inside encoder (Autodesk Fusion 360 design; units mm, degrees)
Autodesk Fusion 360 part; units mm, degrees
note: some values were not read from the file. Set by a fixed rule: which sketch regions a step uses.
(part 1 of 2)
sketch "Sketch1" plane through (0, -20.5, -1.25) normal (0, 0, -1) x (1, 0, 0)
  circle A0 centre (0, -20.5) radius 3
  spline S0 degree 5 poles (-12.6425, -33.7593) (-12.6317, -33.756) (-12.6102, -33.7493) (-12.5779, -33.7393) (-12.535, -33.7257) (-12.4816, -33.7085) (-12.4284, -33.6909) (-12.3754, -33.673) (-12.3227, -33.6548) (-12.2702, -33.6363) (-12.2179, -33.6175) (-12.1659, -33.5983) (-12.114, -33.5788) (-12.0625, -33.5591) (-12.0112, -33.5389) (-11.9601, -33.5185) (-11.9093, -33.4978) (-11.8587, -33.4767) (-11.8084, -33.4553) (-11.7584, -33.4335) (-11.7086, -33.4114) (-11.6591, -33.389) (-11.6099, -33.3662) (-11.561, -33.3431) (-11.5124, -33.3196) (-11.4641, -33.2958) (-11.4161, -33.2716) (-11.3684, -33.2471) (-11.321, -33.2222) (-11.274, -33.1969) (-11.2273, -33.1713) (-11.1809, -33.1453) (-11.1349, -33.1188) (-11.0893, -33.092) (-11.0441, -33.0647) (-10.9992, -33.0371) (-10.9547, -33.009) (-10.9107, -32.9805) (-10.867, -32.9516) (-10.8239, -32.9222) (-10.7812, -32.8923) (-10.739, -32.8619) (-10.6974, -32.8309) (-10.6565, -32.7993) (-10.6161, -32.7671) (-10.5765, -32.7343) (-10.5452, -32.7076) (-10.5221, -32.6872) (-10.5068, -32.6735) (-10.4992, -32.6667) knots -1 -1 -1 -1 -1 -1 -0.977778 -0.955556 -0.933333 -0.911111 -0.888889 -0.866667 -0.844444 -0.822222 -0.8 -0.777778 -0.755556 -0.733333 -0.711111 -0.688889 -0.666667 -0.644444 -0.622222 -0.6 -0.577778 -0.555556 -0.533333 -0.511111 -0.488889 -0.466667 -0.444444 -0.422222 -0.4 -0.377778 -0.355556 -0.333333 -0.311111 -0.288889 -0.266667 -0.244444 -0.222222 -0.2 -0.177778 -0.155556 -0.133333 -0.111111 -0.088889 -0.066667 -0.044444 -0.022222 0 0 0 0 0 0
  arc A1 (-10.4992, -32.6667) -> (-9.4419, -33.5043) centre (0, -20.5) ccw
  spline S1 degree 5 poles (-9.4419, -33.5043) (-9.4469, -33.5133) (-9.4567, -33.5313) (-9.4712, -33.5584) (-9.4901, -33.5949) (-9.513, -33.6411) (-9.5351, -33.6877) (-9.5565, -33.7348) (-9.5772, -33.7824) (-9.5971, -33.8304) (-9.6165, -33.8788) (-9.6352, -33.9275) (-9.6534, -33.9766) (-9.671, -34.026) (-9.6882, -34.0757) (-9.7048, -34.1257) (-9.721, -34.176) (-9.7367, -34.2266) (-9.7519, -34.2774) (-9.7666, -34.3285) (-9.7809, -34.3798) (-9.7947, -34.4314) (-9.8081, -34.4832) (-9.8211, -34.5352) (-9.8337, -34.5875) (-9.8458, -34.64) (-9.8575, -34.6927) (-9.8688, -34.7456) (-9.8797, -34.7987) (-9.8903, -34.852) (-9.9004, -34.9055) (-9.9101, -34.9591) (-9.9194, -35.013) (-9.9284, -35.0671) (-9.937, -35.1213) (-9.9452, -35.1757) (-9.953, -35.2302) (-9.9605, -35.285) (-9.9676, -35.3398) (-9.9743, -35.3949) (-9.9807, -35.4501) (-9.9867, -35.5055) (-9.9923, -35.561) (-9.9976, -35.6166) (-10.0026, -35.6724) (-10.0072, -35.7283) (-10.0106, -35.7732) (-10.0129, -35.8069) (-10.0145, -35.8294) (-10.0152, -35.8407) knots 0 0 0 0 0 0 0.022222 0.044444 0.066667 0.088889 0.111111 0.133333 0.155556 0.177778 0.2 0.222222 0.244444 0.266667 0.288889 0.311111 0.333333 0.355556 0.377778 0.4 0.422222 0.444444 0.466667 0.488889 0.511111 0.533333 0.555556 0.577778 0.6 0.622222 0.644444 0.666667 0.688889 0.711111 0.733333 0.755556 0.777778 0.8 0.822222 0.844444 0.866667 0.888889 0.911111 0.933333 0.955556 0.977778 1 1 1 1 1 1
  arc A2 (-10.0152, -35.8407) -> (-9.6095, -36.098) centre (0, -20.5) ccw
  spline S2 degree 5 poles (-9.6095, -36.098) (-9.5996, -36.0926) (-9.5799, -36.0816) (-9.5504, -36.0651) (-9.5113, -36.0429) (-9.4627, -36.0149) (-9.4143, -35.9866) (-9.3662, -35.9581) (-9.3184, -35.9294) (-9.2709, -35.9003) (-9.2236, -35.8711) (-9.1767, -35.8415) (-9.1301, -35.8117) (-9.0838, -35.7816) (-9.0377, -35.7513) (-8.992, -35.7207) (-8.9466, -35.6898) (-8.9016, -35.6587) (-8.8568, -35.6273) (-8.8124, -35.5956) (-8.7683, -35.5636) (-8.7246, -35.5314) (-8.6812, -35.4989) (-8.6382, -35.4661) (-8.5955, -35.4331) (-8.5532, -35.3997) (-8.5113, -35.3661) (-8.4697, -35.3322) (-8.4286, -35.298) (-8.3878, -35.2635) (-8.3474, -35.2287) (-8.3075, -35.1936) (-8.268, -35.1581) (-8.229, -35.1224) (-8.1904, -35.0864) (-8.1523, -35.05) (-8.1146, -35.0133) (-8.0774, -34.9763) (-8.0407, -34.9389) (-8.0046, -34.9012) (-7.9691, -34.8631) (-7.9341, -34.8245) (-7.8999, -34.7856) (-7.8664, -34.7462) (-7.8337, -34.7063) (-7.8017, -34.6659) (-7.7767, -34.6333) (-7.7583, -34.6086) (-7.7462, -34.592) (-7.7402, -34.5837) knots -1 -1 -1 -1 -1 -1 -0.977778 -0.955556 -0.933333 -0.911111 -0.888889 -0.866667 -0.844444 -0.822222 -0.8 -0.777778 -0.755556 -0.733333 -0.711111 -0.688889 -0.666667 -0.644444 -0.622222 -0.6 -0.577778 -0.555556 -0.533333 -0.511111 -0.488889 -0.466667 -0.444444 -0.422222 -0.4 -0.377778 -0.355556 -0.333333 -0.311111 -0.288889 -0.266667 -0.244444 -0.222222 -0.2 -0.177778 -0.155556 -0.133333 -0.111111 -0.088889 -0.066667 -0.044444 -0.022222 0 0 0 0 0 0
  arc A3 (-7.7402, -34.5837) -> (-6.5319, -35.1832) centre (0, -20.5) ccw
  spline S3 degree 5 poles (-6.5319, -35.1832) (-6.5348, -35.193) (-6.5407, -35.2127) (-6.5493, -35.2422) (-6.5602, -35.2819) (-6.5729, -35.3318) (-6.5849, -35.382) (-6.596, -35.4325) (-6.6063, -35.4833) (-6.6159, -35.5344) (-6.6247, -35.5858) (-6.6329, -35.6374) (-6.6405, -35.6892) (-6.6475, -35.7412) (-6.6539, -35.7934) (-6.6598, -35.8457) (-6.6652, -35.8983) (-6.67, -35.951) (-6.6743, -36.0038) (-6.6781, -36.0569) (-6.6814, -36.1101) (-6.6842, -36.1634) (-6.6865, -36.2169) (-6.6884, -36.2705) (-6.6898, -36.3242) (-6.6908, -36.3781) (-6.6913, -36.432) (-6.6914, -36.4861) (-6.691, -36.5403) (-6.6902, -36.5946) (-6.689, -36.6491) (-6.6873, -36.7036) (-6.6853, -36.7582) (-6.6828, -36.813) (-6.6799, -36.8678) (-6.6766, -36.9227) (-6.6729, -36.9777) (-6.6689, -37.0328) (-6.6644, -37.0879) (-6.6595, -37.1432) (-6.6543, -37.1985) (-6.6486, -37.2539) (-6.6426, -37.3094) (-6.6362, -37.3649) (-6.6295, -37.4205) (-6.6223, -37.4762) (-6.6163, -37.5208) (-6.6117, -37.5542) (-6.6085, -37.5766) (-6.6068, -37.5877) knots 0 0 0 0 0 0 0.022222 0.044444 0.066667 0.088889 0.111111 0.133333 0.155556 0.177778 0.2 0.222222 0.244444 0.266667 0.288889 0.311111 0.333333 0.355556 0.377778 0.4 0.422222 0.444444 0.466667 0.488889 0.511111 0.533333 0.555556 0.577778 0.6 0.622222 0.644444 0.666667 0.688889 0.711111 0.733333 0.755556 0.777778 0.8 0.822222 0.844444 0.866667 0.888889 0.911111 0.933333 0.955556 0.977778 1 1 1 1 1 1
  arc A4 (-6.6068, -37.5877) -> (-6.1565, -37.7551) centre (0, -20.5) ccw
  spline S4 degree 5 poles (-6.1565, -37.7551) (-6.148, -37.7477) (-6.131, -37.7329) (-6.1056, -37.7106) (-6.0719, -37.6807) (-6.0301, -37.6432) (-5.9887, -37.6056) (-5.9476, -37.5677) (-5.9068, -37.5296) (-5.8664, -37.4913) (-5.8263, -37.4529) (-5.7865, -37.4142) (-5.7471, -37.3753) (-5.708, -37.3363) (-5.6693, -37.297) (-5.631, -37.2576) (-5.593, -37.218) (-5.5554, -37.1781) (-5.5181, -37.1381) (-5.4813, -37.0979) (-5.4448, -37.0575) (-5.4087, -37.0169) (-5.3731, -36.9761) (-5.3378, -36.9351) (-5.3029, -36.8938) (-5.2685, -36.8524) (-5.2344, -36.8108) (-5.2009, -36.769) (-5.1677, -36.727) (-5.135, -36.6848) (-5.1028, -36.6423) (-5.071, -36.5997) (-5.0397, -36.5568) (-5.009, -36.5138) (-4.9787, -36.4705) (-4.949, -36.427) (-4.9198, -36.3833) (-4.8911, -36.3393) (-4.863, -36.2951) (-4.8355, -36.2507) (-4.8087, -36.206) (-4.7825, -36.1611) (-4.7571, -36.1159) (-4.7326, -36.0704) (-4.7088, -36.0246) (-4.6859, -35.9784) (-4.6683, -35.9413) (-4.6554, -35.9133) (-4.6471, -35.8946) (-4.6429, -35.8852) knots -1 -1 -1 -1 -1 -1 -0.977778 -0.955556 -0.933333 -0.911111 -0.888889 -0.866667 -0.844444 -0.822222 -0.8 -0.777778 -0.755556 -0.733333 -0.711111 -0.688889 -0.666667 -0.644444 -0.622222 -0.6 -0.577778 -0.555556 -0.533333 -0.511111 -0.488889 -0.466667 -0.444444 -0.422222 -0.4 -0.377778 -0.355556 -0.333333 -0.311111 -0.288889 -0.266667 -0.244444 -0.222222 -0.2 -0.177778 -0.155556 -0.133333 -0.111111 -0.088889 -0.066667 -0.044444 -0.022222 0 0 0 0 0 0
  arc A5 (-4.6429, -35.8852) -> (-3.3363, -36.2204) centre (0, -20.5) ccw
  spline S5 degree 5 poles (-3.3363, -36.2204) (-3.3372, -36.2306) (-3.3389, -36.251) (-3.3411, -36.2818) (-3.3435, -36.3228) (-3.3456, -36.3743) (-3.3469, -36.4258) (-3.3472, -36.4776) (-3.3467, -36.5294) (-3.3455, -36.5814) (-3.3434, -36.6335) (-3.3407, -36.6856) (-3.3373, -36.7379) (-3.3334, -36.7902) (-3.3288, -36.8426) (-3.3237, -36.895) (-3.318, -36.9475) (-3.3118, -37.0001) (-3.305, -37.0527) (-3.2977, -37.1054) (-3.2899, -37.1581) (-3.2815, -37.2108) (-3.2727, -37.2636) (-3.2634, -37.3164) (-3.2536, -37.3693) (-3.2433, -37.4222) (-3.2326, -37.4751) (-3.2214, -37.528) (-3.2098, -37.5809) (-3.1977, -37.6339) (-3.1852, -37.6869) (-3.1723, -37.7399) (-3.1589, -37.7929) (-3.1451, -37.8459) (-3.1309, -37.8989) (-3.1163, -37.952) (-3.1012, -38.005) (-3.0858, -38.058) (-3.0699, -38.1111) (-3.0537, -38.1641) (-3.0371, -38.2171) (-3.02, -38.2701) (-3.0026, -38.3231) (-2.9848, -38.3761) (-2.9666, -38.4291) (-2.9481, -38.4821) (-2.9329, -38.5244) (-2.9214, -38.5562) (-2.9136, -38.5774) (-2.9097, -38.588) knots 0 0 0 0 0 0 0.022222 0.044444 0.066667 0.088889 0.111111 0.133333 0.155556 0.177778 0.2 0.222222 0.244444 0.266667 0.288889 0.311111 0.333333 0.355556 0.377778 0.4 0.422222 0.444444 0.466667 0.488889 0.511111 0.533333 0.555556 0.577778 0.6 0.622222 0.644444 0.666667 0.688889 0.711111 0.733333 0.755556 0.777778 0.8 0.822222 0.844444 0.866667 0.888889 0.911111 0.933333 0.955556 0.977778 1 1 1 1 1 1
  arc A6 (-2.9097, -38.588) -> (-2.4344, -38.658) centre (0, -20.5) ccw
  spline S6 degree 5 poles (-2.4344, -38.658) (-2.4276, -38.649) (-2.4141, -38.631) (-2.3939, -38.6039) (-2.3671, -38.5677) (-2.3341, -38.5224) (-2.3014, -38.4769) (-2.2691, -38.4313) (-2.2371, -38.3856) (-2.2055, -38.3397) (-2.1742, -38.2937) (-2.1434, -38.2477) (-2.1129, -38.2015) (-2.0828, -38.1551) (-2.0531, -38.1087) (-2.0238, -38.0622) (-1.9949, -38.0155) (-1.9664, -37.9687) (-1.9383, -37.9218) (-1.9106, -37.8748) (-1.8833, -37.8277) (-1.8565, -37.7805) (-1.8301, -37.7331) (-1.8041, -37.6857) (-1.7786, -37.6381) (-1.7535, -37.5905) (-1.7288, -37.5427) (-1.7047, -37.4948) (-1.681, -37.4468) (-1.6578, -37.3987) (-1.6351, -37.3505) (-1.6129, -37.3022) (-1.5912, -37.2538) (-1.5701, -37.2053) (-1.5495, -37.1566) (-1.5294, -37.1079) (-1.51, -37.0591) (-1.4911, -37.0101) (-1.4727, -36.961) (-1.4551, -36.9119) (-1.4381, -36.8626) (-1.4219, -36.8132) (-1.4065, -36.7637) (-1.3919, -36.7141) (-1.3782, -36.6643) (-1.3654, -36.6145) (-1.3559, -36.5745) (-1.3491, -36.5444) (-1.3448, -36.5244) (-1.3427, -36.5143) knots -1 -1 -1 -1 -1 -1 -0.977778 -0.955556 -0.933333 -0.911111 -0.888889 -0.866667 -0.844444 -0.822222 -0.8 -0.777778 -0.755556 -0.733333 -0.711111 -0.688889 -0.666667 -0.644444 -0.622222 -0.6 -0.577778 -0.555556 -0.533333 -0.511111 -0.488889 -0.466667 -0.444444 -0.422222 -0.4 -0.377778 -0.355556 -0.333333 -0.311111 -0.288889 -0.266667 -0.244444 -0.222222 -0.2 -0.177778 -0.155556 -0.133333 -0.111111 -0.088889 -0.066667 -0.044444 -0.022222 0 0 0 0 0 0
  arc A7 (-1.3427, -36.5143) -> (0.005, -36.5705) centre (0, -20.5) ccw
  spline S7 degree 5 poles (0.005, -36.5705) (0.0063, -36.5807) (0.0089, -36.601) (0.0132, -36.6315) (0.0193, -36.6722) (0.0279, -36.723) (0.0375, -36.7737) (0.0478, -36.8243) (0.0591, -36.875) (0.0711, -36.9255) (0.084, -36.976) (0.0975, -37.0265) (0.1116, -37.0769) (0.1264, -37.1273) (0.1417, -37.1776) (0.1577, -37.2278) (0.1741, -37.278) (0.1911, -37.3281) (0.2087, -37.3781) (0.2268, -37.4281) (0.2454, -37.4781) (0.2646, -37.5279) (0.2842, -37.5777) (0.3043, -37.6275) (0.3248, -37.6771) (0.3459, -37.7267) (0.3674, -37.7762) (0.3893, -37.8257) (0.4117, -37.875) (0.4345, -37.9243) (0.4577, -37.9736) (0.4814, -38.0227) (0.5055, -38.0718) (0.53, -38.1208) (0.555, -38.1697) (0.5803, -38.2185) (0.606, -38.2672) (0.6322, -38.3159) (0.6587, -38.3645) (0.6856, -38.413) (0.7129, -38.4614) (0.7406, -38.5097) (0.7686, -38.5579) (0.7971, -38.6061) (0.8259, -38.6541) (0.855, -38.7021) (0.8787, -38.7403) (0.8965, -38.769) (0.9085, -38.7881) (0.9146, -38.7977) knots 0 0 0 0 0 0 0.022222 0.044444 0.066667 0.088889 0.111111 0.133333 0.155556 0.177778 0.2 0.222222 0.244444 0.266667 0.288889 0.311111 0.333333 0.355556 0.377778 0.4 0.422222 0.444444 0.466667 0.488889 0.511111 0.533333 0.555556 0.577778 0.6 0.622222 0.644444 0.666667 0.688889 0.711111 0.733333 0.755556 0.777778 0.8 0.822222 0.844444 0.866667 0.888889 0.911111 0.933333 0.955556 0.977778 1 1 1 1 1 1
  arc A8 (0.9146, -38.7977) -> (1.394, -38.7674) centre (0, -20.5) ccw
  spline S8 degree 5 poles (1.394, -38.7674) (1.3988, -38.7572) (1.4083, -38.7367) (1.4224, -38.706) (1.4411, -38.6651) (1.464, -38.6138) (1.4865, -38.5625) (1.5087, -38.5112) (1.5304, -38.4598) (1.5518, -38.4084) (1.5728, -38.357) (1.5934, -38.3055) (1.6136, -38.2539) (1.6334, -38.2024) (1.6528, -38.1508) (1.6718, -38.0992) (1.6904, -38.0475) (1.7085, -37.9958) (1.7263, -37.9441) (1.7436, -37.8924) (1.7605, -37.8406) (1.7769, -37.7888) (1.7929, -37.737) (1.8084, -37.6852) (1.8235, -37.6334) (1.8381, -37.5816) (1.8523, -37.5297) (1.866, -37.4779) (1.8792, -37.426) (1.8919, -37.3741) (1.9041, -37.3222) (1.9158, -37.2704) (1.9269, -37.2185) (1.9375, -37.1666) (1.9475, -37.1148) (1.957, -37.063) (1.9659, -37.0111) (1.9742, -36.9593) (1.9819, -36.9075) (1.9889, -36.8558) (1.9953, -36.804) (2.0009, -36.7524) (2.0057, -36.7007) (2.0096, -36.6492) (2.0127, -36.5976) (2.0148, -36.5462) (2.0158, -36.5051) (2.0162, -36.4743) (2.0163, -36.4538) (2.0162, -36.4435) knots -1 -1 -1 -1 -1 -1 -0.977778 -0.955556 -0.933333 -0.911111 -0.888889 -0.866667 -0.844444 -0.822222 -0.8 -0.777778 -0.755556 -0.733333 -0.711111 -0.688889 -0.666667 -0.644444 -0.622222 -0.6 -0.577778 -0.555556 -0.533333 -0.511111 -0.488889 -0.466667 -0.444444 -0.422222 -0.4 -0.377778 -0.355556 -0.333333 -0.311111 -0.288889 -0.266667 -0.244444 -0.222222 -0.2 -0.177778 -0.155556 -0.133333 -0.111111 -0.088889 -0.066667 -0.044444 -0.022222 0 0 0 0 0 0
  arc A9 (2.0162, -36.4435) -> (3.3462, -36.2183) centre (0, -20.5) ccw
  spline S9 degree 5 poles (3.3462, -36.2183) (3.3495, -36.228) (3.3563, -36.2473) (3.3668, -36.2763) (3.3813, -36.3148) (3.4003, -36.3626) (3.4201, -36.4103) (3.4408, -36.4577) (3.4623, -36.5048) (3.4847, -36.5518) (3.5077, -36.5986) (3.5314, -36.6451) (3.5557, -36.6915) (3.5806, -36.7376) (3.6061, -36.7837) (3.6321, -36.8295) (3.6587, -36.8751) (3.6857, -36.9206) (3.7133, -36.9659) (3.7414, -37.0111) (3.77, -37.056) (3.7991, -37.1008) (3.8286, -37.1455) (3.8586, -37.1899) (3.8891, -37.2342) (3.9199, -37.2783) (3.9513, -37.3223) (3.983, -37.3661) (4.0151, -37.4098) (4.0477, -37.4532) (4.0807, -37.4966) (4.1141, -37.5397) (4.1479, -37.5827) (4.182, -37.6255) (4.2166, -37.6682) (4.2515, -37.7107) (4.2868, -37.753) (4.3225, -37.7952) (4.3585, -37.8372) (4.3949, -37.879) (4.4317, -37.9207) (4.4688, -37.9622) (4.5063, -38.0035) (4.5441, -38.0447) (4.5823, -38.0857) (4.6208, -38.1265) (4.6518, -38.1591) (4.6753, -38.1834) (4.691, -38.1996) (4.6989, -38.2077) knots 0 0 0 0 0 0 0.022222 0.044444 0.066667 0.088889 0.111111 0.133333 0.155556 0.177778 0.2 0.222222 0.244444 0.266667 0.288889 0.311111 0.333333 0.355556 0.377778 0.4 0.422222 0.444444 0.466667 0.488889 0.511111 0.533333 0.555556 0.577778 0.6 0.622222 0.644444 0.666667 0.688889 0.711111 0.733333 0.755556 0.777778 0.8 0.822222 0.844444 0.866667 0.888889 0.911111 0.933333 0.955556 0.977778 1 1 1 1 1 1
  arc A10 (4.6989, -38.2077) -> (5.1616, -38.0784) centre (0, -20.5) ccw
  spline S10 degree 5 poles (5.1616, -38.0784) (5.1641, -38.0674) (5.1692, -38.0454) (5.1766, -38.0124) (5.1863, -37.9685) (5.1981, -37.9136) (5.2094, -37.8588) (5.2204, -37.8039) (5.231, -37.7492) (5.2413, -37.6944) (5.2511, -37.6397) (5.2605, -37.5851) (5.2696, -37.5305) (5.2782, -37.4759) (5.2865, -37.4214) (5.2943, -37.367) (5.3018, -37.3126) (5.3088, -37.2583) (5.3154, -37.204) (5.3216, -37.1498) (5.3273, -37.0957) (5.3326, -37.0416) (5.3375, -36.9876) (5.3419, -36.9337) (5.3459, -36.8799) (5.3494, -36.8261) (5.3525, -36.7725) (5.3551, -36.7189) (5.3572, -36.6654) (5.3589, -36.612) (5.36, -36.5588) (5.3606, -36.5056) (5.3607, -36.4525) (5.3603, -36.3996) (5.3593, -36.3468) (5.3578, -36.2941) (5.3558, -36.2416) (5.3531, -36.1892) (5.3499, -36.1369) (5.346, -36.0848) (5.3415, -36.0329) (5.3362, -35.9812) (5.3302, -35.9297) (5.3233, -35.8784) (5.3156, -35.8274) (5.307, -35.7766) (5.2994, -35.7362) (5.2934, -35.706) (5.2892, -35.686) (5.287, -35.6759) knots -1 -1 -1 -1 -1 -1 -0.977778 -0.955556 -0.933333 -0.911111 -0.888889 -0.866667 -0.844444 -0.822222 -0.8 -0.777778 -0.755556 -0.733333 -0.711111 -0.688889 -0.666667 -0.644444 -0.622222 -0.6 -0.577778 -0.555556 -0.533333 -0.511111 -0.488889 -0.466667 -0.444444 -0.422222 -0.4 -0.377778 -0.355556 -0.333333 -0.311111 -0.288889 -0.266667 -0.244444 -0.222222 -0.2 -0.177778 -0.155556 -0.133333 -0.111111 -0.088889 -0.066667 -0.044444 -0.022222 0 0 0 0 0 0
  arc A11 (5.287, -35.6759) -> (6.5411, -35.1791) centre (0, -20.5) ccw
  spline S11 degree 5 poles (6.5411, -35.1791) (6.5464, -35.1879) (6.557, -35.2054) (6.5733, -35.2315) (6.5955, -35.2662) (6.624, -35.309) (6.6533, -35.3515) (6.6834, -35.3936) (6.7143, -35.4352) (6.7459, -35.4765) (6.7781, -35.5175) (6.811, -35.5581) (6.8444, -35.5984) (6.8784, -35.6384) (6.9129, -35.6781) (6.9478, -35.7175) (6.9833, -35.7566) (7.0192, -35.7955) (7.0556, -35.8341) (7.0925, -35.8724) (7.1298, -35.9104) (7.1676, -35.9482) (7.2057, -35.9857) (7.2443, -36.023) (7.2833, -36.06) (7.3227, -36.0967) (7.3625, -36.1332) (7.4026, -36.1694) (7.4431, -36.2054) (7.484, -36.2412) (7.5253, -36.2767) (7.5669, -36.312) (7.6089, -36.347) (7.6512, -36.3818) (7.6939, -36.4163) (7.7369, -36.4506) (7.7802, -36.4847) (7.8239, -36.5185) (7.8679, -36.5521) (7.9122, -36.5855) (7.9568, -36.6186) (8.0018, -36.6515) (8.047, -36.6841) (8.0926, -36.7165) (8.1384, -36.7487) (8.1846, -36.7806) (8.2217, -36.806) (8.2497, -36.8249) (8.2684, -36.8375) (8.2778, -36.8438) knots 0 0 0 0 0 0 0.022222 0.044444 0.066667 0.088889 0.111111 0.133333 0.155556 0.177778 0.2 0.222222 0.244444 0.266667 0.288889 0.311111 0.333333 0.355556 0.377778 0.4 0.422222 0.444444 0.466667 0.488889 0.511111 0.533333 0.555556 0.577778 0.6 0.622222 0.644444 0.666667 0.688889 0.711111 0.733333 0.755556 0.777778 0.8 0.822222 0.844444 0.866667 0.888889 0.911111 0.933333 0.955556 0.977778 1 1 1 1 1 1
  arc A12 (8.2778, -36.8438) -> (8.7035, -36.6211) centre (0, -20.5) ccw
  spline S12 degree 5 poles (8.7035, -36.6211) (8.7037, -36.6098) (8.7041, -36.5873) (8.7045, -36.5535) (8.7049, -36.5085) (8.705, -36.4523) (8.7047, -36.3963) (8.704, -36.3404) (8.703, -36.2846) (8.7016, -36.229) (8.6999, -36.1734) (8.6978, -36.118) (8.6953, -36.0627) (8.6924, -36.0076) (8.6891, -35.9525) (8.6855, -35.8977) (8.6814, -35.8429) (8.677, -35.7883) (8.6722, -35.7339) (8.667, -35.6796) (8.6613, -35.6254) (8.6553, -35.5714) (8.6488, -35.5176) (8.642, -35.4639) (8.6347, -35.4105) (8.6269, -35.3571) (8.6188, -35.304) (8.6102, -35.2511) (8.6011, -35.1983) (8.5917, -35.1458) (8.5817, -35.0934) (8.5713, -35.0413) (8.5603, -34.9894) (8.5489, -34.9377) (8.537, -34.8863) (8.5245, -34.8351) (8.5116, -34.7841) (8.4981, -34.7334) (8.4841, -34.6829) (8.4695, -34.6328) (8.4542, -34.5829) (8.4383, -34.5334) (8.4217, -34.4843) (8.4043, -34.4356) (8.3862, -34.3873) (8.3672, -34.3394) (8.3514, -34.3015) (8.3392, -34.2732) (8.3309, -34.2544) (8.3267, -34.2451) knots -1 -1 -1 -1 -1 -1 -0.977778 -0.955556 -0.933333 -0.911111 -0.888889 -0.866667 -0.844444 -0.822222 -0.8 -0.777778 -0.755556 -0.733333 -0.711111 -0.688889 -0.666667 -0.644444 -0.622222 -0.6 -0.577778 -0.555556 -0.533333 -0.511111 -0.488889 -0.466667 -0.444444 -0.422222 -0.4 -0.377778 -0.355556 -0.333333 -0.311111 -0.288889 -0.266667 -0.244444 -0.222222 -0.2 -0.177778 -0.155556 -0.133333 -0.111111 -0.088889 -0.066667 -0.044444 -0.022222 0 0 0 0 0 0
  arc A13 (8.3267, -34.2451) -> (9.4501, -33.4984) centre (0, -20.5) ccw
  spline S13 degree 5 poles (9.4501, -33.4984) (9.4571, -33.5058) (9.4712, -33.5208) (9.4925, -33.543) (9.5214, -33.5722) (9.5582, -33.6082) (9.5957, -33.6437) (9.6339, -33.6785) (9.6728, -33.7129) (9.7122, -33.7467) (9.7523, -33.7801) (9.7929, -33.8129) (9.834, -33.8454) (9.8755, -33.8775) (9.9175, -33.9091) (9.9599, -33.9404) (10.0027, -33.9713) (10.0459, -34.0019) (10.0896, -34.032) (10.1336, -34.0618) (10.178, -34.0913) (10.2228, -34.1204) (10.2679, -34.1491) (10.3134, -34.1776) (10.3593, -34.2056) (10.4054, -34.2334) (10.4519, -34.2608) (10.4987, -34.2879) (10.5458, -34.3147) (10.5933, -34.3412) (10.641, -34.3674) (10.6891, -34.3932) (10.7374, -34.4187) (10.786, -34.4439) (10.835, -34.4689) (10.8842, -34.4935) (10.9336, -34.5178) (10.9834, -34.5418) (11.0334, -34.5655) (11.0837, -34.5889) (11.1342, -34.612) (11.185, -34.6348) (11.236, -34.6574) (11.2873, -34.6796) (11.3389, -34.7015) (11.3906, -34.7232) (11.4323, -34.7403) (11.4636, -34.753) (11.4845, -34.7614) (11.495, -34.7656) knots 0 0 0 0 0 0 0.022222 0.044444 0.066667 0.088889 0.111111 0.133333 0.155556 0.177778 0.2 0.222222 0.244444 0.266667 0.288889 0.311111 0.333333 0.355556 0.377778 0.4 0.422222 0.444444 0.466667 0.488889 0.511111 0.533333 0.555556 0.577778 0.6 0.622222 0.644444 0.666667 0.688889 0.711111 0.733333 0.755556 0.777778 0.8 0.822222 0.844444 0.866667 0.888889 0.911111 0.933333 0.955556 0.977778 1 1 1 1 1 1
  arc A14 (11.495, -34.7656) -> (11.8651, -34.4592) centre (0, -20.5) ccw
  spline S14 degree 5 poles (11.8651, -34.4592) (11.863, -34.4482) (11.8586, -34.426) (11.852, -34.3929) (11.843, -34.3488) (11.8314, -34.2939) (11.8195, -34.2391) (11.8072, -34.1846) (11.7947, -34.1302) (11.7817, -34.0761) (11.7685, -34.0221) (11.7549, -33.9684) (11.7409, -33.9148) (11.7266, -33.8614) (11.712, -33.8083) (11.697, -33.7554) (11.6817, -33.7027) (11.666, -33.6502) (11.65, -33.5979) (11.6336, -33.5459) (11.6168, -33.4941) (11.5997, -33.4425) (11.5822, -33.3912) (11.5643, -33.3402) (11.546, -33.2894) (11.5274, -33.2388) (11.5084, -33.1886) (11.489, -33.1386) (11.4691, -33.0889) (11.4489, -33.0394) (11.4283, -32.9903) (11.4073, -32.9415) (11.3858, -32.893) (11.3639, -32.8448) (11.3415, -32.7969) (11.3187, -32.7494) (11.2954, -32.7023) (11.2717, -32.6555) (11.2475, -32.6091) (11.2228, -32.563) (11.1975, -32.5174) (11.1717, -32.4723) (11.1452, -32.4278) (11.1181, -32.3837) (11.0903, -32.3403) (11.0618, -32.2974) (11.0384, -32.2635) (11.0206, -32.2384) (11.0086, -32.2218) (11.0025, -32.2135) knots -1 -1 -1 -1 -1 -1 -0.977778 -0.955556 -0.933333 -0.911111 -0.888889 -0.866667 -0.844444 -0.822222 -0.8 -0.777778 -0.755556 -0.733333 -0.711111 -0.688889 -0.666667 -0.644444 -0.622222 -0.6 -0.577778 -0.555556 -0.533333 -0.511111 -0.488889 -0.466667 -0.444444 -0.422222 -0.4 -0.377778 -0.355556 -0.333333 -0.311111 -0.288889 -0.266667 -0.244444 -0.222222 -0.2 -0.177778 -0.155556 -0.133333 -0.111111 -0.088889 -0.066667 -0.044444 -0.022222 0 0 0 0 0 0
  arc A15 (11.0025, -32.2135) -> (11.9461, -31.2495) centre (0, -20.5) ccw
  spline S15 degree 5 poles (11.9461, -31.2495) (11.9545, -31.2554) (11.9714, -31.2671) (11.9969, -31.2843) (12.0312, -31.3069) (12.0747, -31.3345) (12.1188, -31.3614) (12.1634, -31.3876) (12.2085, -31.4131) (12.2542, -31.438) (12.3003, -31.4622) (12.3468, -31.486) (12.3937, -31.5092) (12.441, -31.5319) (12.4887, -31.5541) (12.5367, -31.5759) (12.585, -31.5973) (12.6336, -31.6181) (12.6826, -31.6386) (12.7318, -31.6586) (12.7814, -31.6782) (12.8312, -31.6973) (12.8814, -31.716) (12.9318, -31.7344) (12.9824, -31.7523) (13.0334, -31.7699) (13.0845, -31.7871) (13.136, -31.8038) (13.1876, -31.8202) (13.2395, -31.8363) (13.2917, -31.8519) (13.344, -31.8672) (13.3966, -31.8821) (13.4495, -31.8967) (13.5025, -31.9109) (13.5557, -31.9247) (13.6092, -31.9382) (13.6628, -31.9514) (13.7167, -31.9642) (13.7707, -31.9766) (13.8249, -31.9887) (13.8794, -32.0005) (13.934, -32.0119) (13.9888, -32.023) (14.0437, -32.0337) (14.0989, -32.0441) (14.1432, -32.0522) (14.1764, -32.0581) (14.1987, -32.062) (14.2098, -32.0639) knots 0 0 0 0 0 0 0.022222 0.044444 0.066667 0.088889 0.111111 0.133333 0.155556 0.177778 0.2 0.222222 0.244444 0.266667 0.288889 0.311111 0.333333 0.355556 0.377778 0.4 0.422222 0.444444 0.466667 0.488889 0.511111 0.533333 0.555556 0.577778 0.6 0.622222 0.644444 0.666667 0.688889 0.711111 0.733333 0.755556 0.777778 0.8 0.822222 0.844444 0.866667 0.888889 0.911111 0.933333 0.955556 0.977778 1 1 1 1 1 1
  arc A16 (14.2098, -32.0639) -> (14.5081, -31.6873) centre (0, -20.5) ccw
  spline S16 degree 5 poles (14.5081, -31.6873) (14.5037, -31.6769) (14.4949, -31.6562) (14.4815, -31.6251) (14.4635, -31.5839) (14.4408, -31.5326) (14.4177, -31.4815) (14.3944, -31.4307) (14.3708, -31.3801) (14.3469, -31.3299) (14.3227, -31.2798) (14.2982, -31.2301) (14.2735, -31.1806) (14.2484, -31.1314) (14.223, -31.0824) (14.1974, -31.0338) (14.1714, -30.9854) (14.1452, -30.9373) (14.1186, -30.8895) (14.0917, -30.842) (14.0646, -30.7949) (14.0371, -30.748) (14.0093, -30.7015) (13.9812, -30.6552) (13.9528, -30.6093) (13.924, -30.5638) (13.895, -30.5186) (13.8656, -30.4737) (13.8359, -30.4292) (13.8058, -30.385) (13.7754, -30.3413) (13.7447, -30.2979) (13.7136, -30.2549) (13.6821, -30.2123) (13.6503, -30.1702) (13.6181, -30.1285) (13.5856, -30.0872) (13.5526, -30.0463) (13.5193, -30.006) (13.4856, -29.9661) (13.4514, -29.9267) (13.4167, -29.888) (13.3816, -29.8499) (13.3459, -29.8125) (13.3096, -29.7757) (13.2728, -29.7397) (13.243, -29.7114) (13.2203, -29.6906) (13.2051, -29.6768) (13.1975, -29.6699) knots -1 -1 -1 -1 -1 -1 -0.977778 -0.955556 -0.933333 -0.911111 -0.888889 -0.866667 -0.844444 -0.822222 -0.8 -0.777778 -0.755556 -0.733333 -0.711111 -0.688889 -0.666667 -0.644444 -0.622222 -0.6 -0.577778 -0.555556 -0.533333 -0.511111 -0.488889 -0.466667 -0.444444 -0.422222 -0.4 -0.377778 -0.355556 -0.333333 -0.311111 -0.288889 -0.266667 -0.244444 -0.222222 -0.2 -0.177778 -0.155556 -0.133333 -0.111111 -0.088889 -0.066667 -0.044444 -0.022222 0 0 0 0 0 0
  arc A17 (13.1975, -29.6699) -> (13.92, -28.5309) centre (0, -20.5) ccw
  spline S17 degree 5 poles (13.92, -28.5309) (13.9294, -28.5349) (13.9484, -28.5428) (13.9769, -28.5544) (14.0152, -28.5694) (14.0635, -28.5873) (14.1121, -28.6044) (14.1612, -28.6207) (14.2107, -28.6363) (14.2605, -28.6512) (14.3107, -28.6653) (14.3611, -28.6788) (14.4118, -28.6918) (14.4628, -28.7042) (14.5141, -28.716) (14.5655, -28.7274) (14.6172, -28.7382) (14.6691, -28.7485) (14.7213, -28.7583) (14.7736, -28.7677) (14.8262, -28.7765) (14.8789, -28.7849) (14.9318, -28.7928) (14.9849, -28.8002) (15.0382, -28.8072) (15.0917, -28.8138) (15.1453, -28.82) (15.1991, -28.8257) (15.2531, -28.831) (15.3072, -28.8359) (15.3614, -28.8404) (15.4158, -28.8444) (15.4704, -28.8481) (15.5251, -28.8513) (15.5799, -28.8542) (15.6348, -28.8567) (15.6899, -28.8588) (15.7451, -28.8605) (15.8004, -28.8618) (15.8559, -28.8627) (15.9115, -28.8633) (15.9671, -28.8635) (16.0229, -28.8633) (16.0788, -28.8628) (16.1348, -28.8618) (16.191, -28.8606) (16.2359, -28.8592) (16.2697, -28.8581) (16.2922, -28.8572) (16.3035, -28.8568) knots 0 0 0 0 0 0 0.022222 0.044444 0.066667 0.088889 0.111111 0.133333 0.155556 0.177778 0.2 0.222222 0.244444 0.266667 0.288889 0.311111 0.333333 0.355556 0.377778 0.4 0.422222 0.444444 0.466667 0.488889 0.511111 0.533333 0.555556 0.577778 0.6 0.622222 0.644444 0.666667 0.688889 0.711111 0.733333 0.755556 0.777778 0.8 0.822222 0.844444 0.866667 0.888889 0.911111 0.933333 0.955556 0.977778 1 1 1 1 1 1
  arc A18 (16.3035, -28.8568) -> (16.5171, -28.4264) centre (0, -20.5) ccw
  spline S18 degree 5 poles (16.5171, -28.4264) (16.5106, -28.4172) (16.4976, -28.3987) (16.4781, -28.3711) (16.4519, -28.3345) (16.419, -28.2891) (16.3859, -28.2439) (16.3525, -28.1991) (16.3189, -28.1545) (16.285, -28.1103) (16.251, -28.0664) (16.2167, -28.0228) (16.1822, -27.9796) (16.1474, -27.9366) (16.1124, -27.894) (16.0772, -27.8518) (16.0418, -27.8099) (16.0061, -27.7683) (15.9702, -27.7271) (15.934, -27.6862) (15.8976, -27.6457) (15.861, -27.6056) (15.8242, -27.5658) (15.7871, -27.5265) (15.7497, -27.4875) (15.7121, -27.4489) (15.6743, -27.4107) (15.6362, -27.3729) (15.5979, -27.3356) (15.5594, -27.2986) (15.5205, -27.2621) (15.4814, -27.2261) (15.4421, -27.1905) (15.4025, -27.1554) (15.3626, -27.1208) (15.3224, -27.0867) (15.282, -27.0531) (15.2413, -27.02) (15.2003, -26.9874) (15.159, -26.9554) (15.1174, -26.924) (15.0754, -26.8934) (15.0331, -26.8634) (14.9904, -26.8342) (14.9473, -26.8058) (14.9038, -26.7782) (14.8687, -26.7568) (14.8422, -26.7411) (14.8245, -26.7308) (14.8156, -26.7257) knots -1 -1 -1 -1 -1 -1 -0.977778 -0.955556 -0.933333 -0.911111 -0.888889 -0.866667 -0.844444 -0.822222 -0.8 -0.777778 -0.755556 -0.733333 -0.711111 -0.688889 -0.666667 -0.644444 -0.622222 -0.6 -0.577778 -0.555556 -0.533333 -0.511111 -0.488889 -0.466667 -0.444444 -0.422222 -0.4 -0.377778 -0.355556 -0.333333 -0.311111 -0.288889 -0.266667 -0.244444 -0.222222 -0.2 -0.177778 -0.155556 -0.133333 -0.111111 -0.088889 -0.066667 -0.044444 -0.022222 0 0 0 0 0 0
  arc A19 (14.8156, -26.7257) -> (15.2855, -25.4613) centre (0, -20.5) ccw
  spline S19 degree 5 poles (15.2855, -25.4613) (15.2956, -25.4632) (15.3158, -25.467) (15.3461, -25.4724) (15.3866, -25.4791) (15.4376, -25.4866) (15.4888, -25.4932) (15.5402, -25.499) (15.5918, -25.5039) (15.6436, -25.5081) (15.6956, -25.5115) (15.7478, -25.5143) (15.8001, -25.5164) (15.8525, -25.5179) (15.9051, -25.5188) (15.9578, -25.5192) (16.0106, -25.5191) (16.0635, -25.5184) (16.1166, -25.5171) (16.1697, -25.5154) (16.2229, -25.5131) (16.2763, -25.5103) (16.3297, -25.507) (16.3832, -25.5033) (16.4368, -25.4991) (16.4904, -25.4944) (16.5442, -25.4893) (16.598, -25.4837) (16.6519, -25.4777) (16.7058, -25.4712) (16.7598, -25.4643) (16.8139, -25.4569) (16.868, -25.4492) (16.9221, -25.441) (16.9764, -25.4324) (17.0306, -25.4234) (17.0849, -25.414) (17.1393, -25.4042) (17.1937, -25.394) (17.2481, -25.3834) (17.3026, -25.3724) (17.3571, -25.361) (17.4116, -25.3492) (17.4662, -25.337) (17.5208, -25.3245) (17.5754, -25.3116) (17.6191, -25.3009) (17.6519, -25.2928) (17.6738, -25.2873) (17.6847, -25.2845) knots 0 0 0 0 0 0 0.022222 0.044444 0.066667 0.088889 0.111111 0.133333 0.155556 0.177778 0.2 0.222222 0.244444 0.266667 0.288889 0.311111 0.333333 0.355556 0.377778 0.4 0.422222 0.444444 0.466667 0.488889 0.511111 0.533333 0.555556 0.577778 0.6 0.622222 0.644444 0.666667 0.688889 0.711111 0.733333 0.755556 0.777778 0.8 0.822222 0.844444 0.866667 0.888889 0.911111 0.933333 0.955556 0.977778 1 1 1 1 1 1
  arc A20 (17.6847, -25.2845) -> (17.8041, -24.8191) centre (0, -20.5) ccw
  spline S20 degree 5 poles (17.8041, -24.8191) (17.7959, -24.8114) (17.7793, -24.7961) (17.7545, -24.7731) (17.7213, -24.7428) (17.6797, -24.7052) (17.6378, -24.6679) (17.5959, -24.631) (17.5537, -24.5944) (17.5114, -24.5582) (17.469, -24.5223) (17.4264, -24.4868) (17.3836, -24.4516) (17.3407, -24.4169) (17.2976, -24.3825) (17.2544, -24.3485) (17.211, -24.3148) (17.1675, -24.2816) (17.1238, -24.2488) (17.0799, -24.2163) (17.0359, -24.1843) (16.9918, -24.1526) (16.9474, -24.1214) (16.903, -24.0906) (16.8583, -24.0602) (16.8136, -24.0303) (16.7686, -24.0008) (16.7235, -23.9718) (16.6783, -23.9432) (16.6329, -23.9151) (16.5873, -23.8875) (16.5416, -23.8603) (16.4957, -23.8337) (16.4496, -23.8076) (16.4034, -23.7821) (16.357, -23.7571) (16.3105, -23.7326) (16.2638, -23.7087) (16.2169, -23.6853) (16.1699, -23.6626) (16.1227, -23.6406) (16.0752, -23.6193) (16.0276, -23.5988) (15.9798, -23.5791) (15.9317, -23.5603) (15.8835, -23.5423) (15.8447, -23.5287) (15.8155, -23.5188) (15.796, -23.5124) (15.7862, -23.5093) knots -1 -1 -1 -1 -1 -1 -0.977778 -0.955556 -0.933333 -0.911111 -0.888889 -0.866667 -0.844444 -0.822222 -0.8 -0.777778 -0.755556 -0.733333 -0.711111 -0.688889 -0.666667 -0.644444 -0.622222 -0.6 -0.577778 -0.555556 -0.533333 -0.511111 -0.488889 -0.466667 -0.444444 -0.422222 -0.4 -0.377778 -0.355556 -0.333333 -0.311111 -0.288889 -0.266667 -0.244444 -0.222222 -0.2 -0.177778 -0.155556 -0.133333 -0.111111 -0.088889 -0.066667 -0.044444 -0.022222 0 0 0 0 0 0
  arc A21 (15.7862, -23.5093) -> (15.983, -22.1748) centre (0, -20.5) ccw
  spline S21 degree 5 poles (15.983, -22.1748) (15.9933, -22.1746) (16.0138, -22.1741) (16.0445, -22.1731) (16.0856, -22.1712) (16.137, -22.168) (16.1884, -22.1638) (16.2399, -22.1588) (16.2914, -22.1529) (16.343, -22.1462) (16.3946, -22.1387) (16.4462, -22.1306) (16.4978, -22.1217) (16.5494, -22.1123) (16.601, -22.1023) (16.6526, -22.0917) (16.7043, -22.0806) (16.7559, -22.0689) (16.8075, -22.0567) (16.8591, -22.0439) (16.9107, -22.0306) (16.9623, -22.0168) (17.0139, -22.0025) (17.0654, -21.9877) (17.117, -21.9724) (17.1685, -21.9567) (17.22, -21.9405) (17.2714, -21.9239) (17.3229, -21.9068) (17.3743, -21.8892) (17.4257, -21.8712) (17.477, -21.8528) (17.5284, -21.834) (17.5796, -21.8147) (17.6309, -21.795) (17.6821, -21.775) (17.7333, -21.7545) (17.7844, -21.7336) (17.8355, -21.7123) (17.8865, -21.6906) (17.9375, -21.6685) (17.9885, -21.646) (18.0393, -21.6231) (18.0902, -21.5999) (18.141, -21.5763) (18.1917, -21.5523) (18.2323, -21.5328) (18.2627, -21.518) (18.2829, -21.5081) (18.293, -21.5031) knots 0 0 0 0 0 0 0.022222 0.044444 0.066667 0.088889 0.111111 0.133333 0.155556 0.177778 0.2 0.222222 0.244444 0.266667 0.288889 0.311111 0.333333 0.355556 0.377778 0.4 0.422222 0.444444 0.466667 0.488889 0.511111 0.533333 0.555556 0.577778 0.6 0.622222 0.644444 0.666667 0.688889 0.711111 0.733333 0.755556 0.777778 0.8 0.822222 0.844444 0.866667 0.888889 0.911111 0.933333 0.955556 0.977778 1 1 1 1 1 1
  arc A22 (18.293, -21.5031) -> (18.313, -21.023) centre (0, -20.5) ccw
  spline S22 degree 5 poles (18.313, -21.023) (18.3034, -21.0172) (18.284, -21.0057) (18.255, -20.9884) (18.2162, -20.9656) (18.1676, -20.9375) (18.119, -20.9097) (18.0702, -20.8823) (18.0214, -20.8553) (17.9725, -20.8286) (17.9235, -20.8024) (17.8745, -20.7765) (17.8254, -20.751) (17.7761, -20.726) (17.7269, -20.7013) (17.6775, -20.677) (17.6281, -20.6531) (17.5786, -20.6296) (17.529, -20.6066) (17.4794, -20.584) (17.4296, -20.5618) (17.3799, -20.54) (17.33, -20.5187) (17.2801, -20.4978) (17.2302, -20.4774) (17.1801, -20.4574) (17.13, -20.4379) (17.0799, -20.4189) (17.0297, -20.4004) (16.9794, -20.3823) (16.9291, -20.3647) (16.8788, -20.3477) (16.8283, -20.3312) (16.7779, -20.3153) (16.7273, -20.2999) (16.6768, -20.2851) (16.6262, -20.2708) (16.5755, -20.2571) (16.5248, -20.244) (16.4741, -20.2316) (16.4233, -20.2199) (16.3725, -20.2089) (16.3216, -20.1987) (16.2708, -20.1894) (16.2198, -20.181) (16.1689, -20.1735) (16.1281, -20.1682) (16.0975, -20.1646) (16.0771, -20.1624) (16.0669, -20.1614) knots -1 -1 -1 -1 -1 -1 -0.977778 -0.955556 -0.933333 -0.911111 -0.888889 -0.866667 -0.844444 -0.822222 -0.8 -0.777778 -0.755556 -0.733333 -0.711111 -0.688889 -0.666667 -0.644444 -0.622222 -0.6 -0.577778 -0.555556 -0.533333 -0.511111 -0.488889 -0.466667 -0.444444 -0.422222 -0.4 -0.377778 -0.355556 -0.333333 -0.311111 -0.288889 -0.266667 -0.244444 -0.222222 -0.2 -0.177778 -0.155556 -0.133333 -0.111111 -0.088889 -0.066667 -0.044444 -0.022222 0 0 0 0 0 0
  arc A23 (16.0669, -20.1614) -> (15.9819, -18.8152) centre (0, -20.5) ccw
  spline S23 degree 5 poles (15.9819, -18.8152) (15.9919, -18.8128) (16.0119, -18.8081) (16.0418, -18.8007) (16.0816, -18.7903) (16.1312, -18.7764) (16.1806, -18.7617) (16.2299, -18.7461) (16.2791, -18.7296) (16.3281, -18.7123) (16.377, -18.6943) (16.4258, -18.6756) (16.4744, -18.6562) (16.523, -18.6363) (16.5714, -18.6158) (16.6197, -18.5947) (16.6679, -18.5731) (16.7159, -18.5509) (16.7639, -18.5282) (16.8117, -18.505) (16.8594, -18.4812) (16.907, -18.457) (16.9545, -18.4323) (17.0018, -18.4071) (17.0491, -18.3814) (17.0962, -18.3553) (17.1432, -18.3288) (17.1901, -18.3018) (17.2368, -18.2744) (17.2835, -18.2465) (17.33, -18.2183) (17.3764, -18.1896) (17.4227, -18.1605) (17.4688, -18.131) (17.5149, -18.1011) (17.5608, -18.0708) (17.6066, -18.0401) (17.6522, -18.009) (17.6978, -17.9776) (17.7432, -17.9457) (17.7885, -17.9135) (17.8336, -17.8809) (17.8787, -17.848) (17.9236, -17.8147) (17.9683, -17.781) (18.013, -17.747) (18.0486, -17.7195) (18.0752, -17.6987) (18.093, -17.6848) (18.1018, -17.6778) knots 0 0 0 0 0 0 0.022222 0.044444 0.066667 0.088889 0.111111 0.133333 0.155556 0.177778 0.2 0.222222 0.244444 0.266667 0.288889 0.311111 0.333333 0.355556 0.377778 0.4 0.422222 0.444444 0.466667 0.488889 0.511111 0.533333 0.555556 0.577778 0.6 0.622222 0.644444 0.666667 0.688889 0.711111 0.733333 0.755556 0.777778 0.8 0.822222 0.844444 0.866667 0.888889 0.911111 0.933333 0.955556 0.977778 1 1 1 1 1 1
  arc A24 (18.1018, -17.6778) -> (18.0216, -17.2041) centre (0, -20.5) ccw
  spline S24 degree 5 poles (18.0216, -17.2041) (18.0109, -17.2005) (17.9896, -17.1931) (17.9576, -17.1823) (17.9149, -17.1681) (17.8616, -17.1506) (17.8082, -17.1336) (17.7548, -17.1169) (17.7015, -17.1007) (17.6481, -17.0848) (17.5947, -17.0693) (17.5414, -17.0542) (17.488, -17.0395) (17.4347, -17.0251) (17.3813, -17.0112) (17.328, -16.9978) (17.2747, -16.9847) (17.2214, -16.972) (17.1681, -16.9598) (17.1148, -16.948) (17.0616, -16.9366) (17.0084, -16.9257) (16.9552, -16.9152) (16.9021, -16.9051) (16.8489, -16.8955) (16.7959, -16.8864) (16.7428, -16.8778) (16.6898, -16.8696) (16.6368, -16.8619) (16.5839, -16.8546) (16.5311, -16.8479) (16.4783, -16.8418) (16.4255, -16.8361) (16.3728, -16.831) (16.3202, -16.8265) (16.2677, -16.8225) (16.2152, -16.819) (16.1628, -16.8162) (16.1105, -16.8139) (16.0583, -16.8123) (16.0062, -16.8114) (15.9542, -16.8112) (15.9023, -16.8119) (15.8506, -16.8133) (15.7991, -16.8157) (15.7477, -16.8189) (15.7067, -16.8222) (15.676, -16.8251) (15.6556, -16.8272) (15.6454, -16.8283) knots -1 -1 -1 -1 -1 -1 -0.977778 -0.955556 -0.933333 -0.911111 -0.888889 -0.866667 -0.844444 -0.822222 -0.8 -0.777778 -0.755556 -0.733333 -0.711111 -0.688889 -0.666667 -0.644444 -0.622222 -0.6 -0.577778 -0.555556 -0.533333 -0.511111 -0.488889 -0.466667 -0.444444 -0.422222 -0.4 -0.377778 -0.355556 -0.333333 -0.311111 -0.288889 -0.266667 -0.244444 -0.222222 -0.2 -0.177778 -0.155556 -0.133333 -0.111111 -0.088889 -0.066667 -0.044444 -0.022222 0 0 0 0 0 0
  arc A25 (15.6454, -16.8283) -> (15.2824, -15.5292) centre (0, -20.5) ccw
  spline S25 degree 5 poles (15.2824, -15.5292) (15.2917, -15.5248) (15.3102, -15.516) (15.3379, -15.5026) (15.3747, -15.4841) (15.4203, -15.4603) (15.4656, -15.4355) (15.5106, -15.41) (15.5553, -15.3837) (15.5996, -15.3566) (15.6437, -15.3288) (15.6875, -15.3003) (15.7311, -15.2713) (15.7744, -15.2417) (15.8175, -15.2115) (15.8604, -15.1809) (15.903, -15.1497) (15.9454, -15.118) (15.9876, -15.0859) (16.0295, -15.0532) (16.0713, -15.0201) (16.1128, -14.9865) (16.1541, -14.9524) (16.1952, -14.9179) (16.236, -14.883) (16.2767, -14.8477) (16.3171, -14.812) (16.3574, -14.7758) (16.3974, -14.7393) (16.4373, -14.7024) (16.4769, -14.665) (16.5163, -14.6273) (16.5555, -14.5892) (16.5945, -14.5508) (16.6334, -14.512) (16.672, -14.4728) (16.7104, -14.4332) (16.7486, -14.3934) (16.7866, -14.3531) (16.8244, -14.3125) (16.862, -14.2716) (16.8994, -14.2304) (16.9366, -14.1888) (16.9736, -14.1469) (17.0104, -14.1046) (17.047, -14.0621) (17.0761, -14.0278) (17.0978, -14.0019) (17.1123, -13.9846) (17.1195, -13.9759) knots 0 0 0 0 0 0 0.022222 0.044444 0.066667 0.088889 0.111111 0.133333 0.155556 0.177778 0.2 0.222222 0.244444 0.266667 0.288889 0.311111 0.333333 0.355556 0.377778 0.4 0.422222 0.444444 0.466667 0.488889 0.511111 0.533333 0.555556 0.577778 0.6 0.622222 0.644444 0.666667 0.688889 0.711111 0.733333 0.755556 0.777778 0.8 0.822222 0.844444 0.866667 0.888889 0.911111 0.933333 0.955556 0.977778 1 1 1 1 1 1
  arc A26 (17.1195, -13.9759) -> (16.9425, -13.5292) centre (0, -20.5) ccw
  spline S26 degree 5 poles (16.9425, -13.5292) (16.9313, -13.5279) (16.9089, -13.5252) (16.8754, -13.5212) (16.8307, -13.5161) (16.7749, -13.5102) (16.7191, -13.5046) (16.6635, -13.4994) (16.6079, -13.4946) (16.5524, -13.4901) (16.497, -13.4861) (16.4416, -13.4824) (16.3864, -13.4791) (16.3312, -13.4762) (16.2762, -13.4737) (16.2212, -13.4716) (16.1663, -13.4699) (16.1116, -13.4686) (16.0569, -13.4677) (16.0023, -13.4672) (15.9479, -13.4672) (15.8936, -13.4675) (15.8394, -13.4683) (15.7853, -13.4695) (15.7313, -13.4712) (15.6775, -13.4733) (15.6238, -13.4759) (15.5703, -13.4789) (15.5169, -13.4824) (15.4636, -13.4863) (15.4105, -13.4907) (15.3576, -13.4957) (15.3048, -13.5011) (15.2522, -13.5071) (15.1998, -13.5136) (15.1476, -13.5206) (15.0955, -13.5281) (15.0437, -13.5362) (14.9921, -13.5449) (14.9407, -13.5542) (14.8895, -13.5641) (14.8386, -13.5748) (14.788, -13.5862) (14.7378, -13.5984) (14.6878, -13.6114) (14.6382, -13.6252) (14.5988, -13.637) (14.5694, -13.6462) (14.5499, -13.6524) (14.5401, -13.6556) knots -1 -1 -1 -1 -1 -1 -0.977778 -0.955556 -0.933333 -0.911111 -0.888889 -0.866667 -0.844444 -0.822222 -0.8 -0.777778 -0.755556 -0.733333 -0.711111 -0.688889 -0.666667 -0.644444 -0.622222 -0.6 -0.577778 -0.555556 -0.533333 -0.511111 -0.488889 -0.466667 -0.444444 -0.422222 -0.4 -0.377778 -0.355556 -0.333333 -0.311111 -0.288889 -0.266667 -0.244444 -0.222222 -0.2 -0.177778 -0.155556 -0.133333 -0.111111 -0.088889 -0.066667 -0.044444 -0.022222 0 0 0 0 0 0
  arc A27 (14.5401, -13.6556) -> (13.915, -12.4604) centre (0, -20.5) ccw
  spline S27 degree 5 poles (13.915, -12.4604) (13.9231, -12.4542) (13.9394, -12.4417) (13.9637, -12.4228) (13.9959, -12.3972) (14.0355, -12.3643) (14.0747, -12.3307) (14.1134, -12.2964) (14.1516, -12.2613) (14.1894, -12.2256) (14.2267, -12.1893) (14.2636, -12.1523) (14.3002, -12.1149) (14.3364, -12.0769) (14.3723, -12.0385) (14.4079, -11.9996) (14.4431, -11.9602) (14.478, -11.9204) (14.5126, -11.8802) (14.5468, -11.8395) (14.5807, -11.7984) (14.6143, -11.7569) (14.6477, -11.715) (14.6807, -11.6728) (14.7134, -11.6301) (14.7458, -11.5871) (14.778, -11.5438) (14.8098, -11.5) (14.8414, -11.456) (14.8727, -11.4115) (14.9037, -11.3668) (14.9344, -11.3217) (14.9648, -11.2763) (14.995, -11.2306) (15.0249, -11.1845) (15.0545, -11.1382) (15.0839, -11.0915) (15.1129, -11.0446) (15.1418, -10.9973) (15.1703, -10.9498) (15.1986, -10.9019) (15.2266, -10.8538) (15.2543, -10.8054) (15.2818, -10.7567) (15.309, -10.7077) (15.3359, -10.6585) (15.3573, -10.6189) (15.3732, -10.5891) (15.3837, -10.5691) (15.389, -10.5591) knots 0 0 0 0 0 0 0.022222 0.044444 0.066667 0.088889 0.111111 0.133333 0.155556 0.177778 0.2 0.222222 0.244444 0.266667 0.288889 0.311111 0.333333 0.355556 0.377778 0.4 0.422222 0.444444 0.466667 0.488889 0.511111 0.533333 0.555556 0.577778 0.6 0.622222 0.644444 0.666667 0.688889 0.711111 0.733333 0.755556 0.777778 0.8 0.822222 0.844444 0.866667 0.888889 0.911111 0.933333 0.955556 0.977778 1 1 1 1 1 1
  arc A28 (15.389, -10.5591) -> (15.123, -10.159) centre (0, -20.5) ccw
  spline S28 degree 5 poles (15.123, -10.159) (15.1118, -10.16) (15.0893, -10.162) (15.0556, -10.1651) (15.0109, -10.1695) (14.955, -10.1753) (14.8994, -10.1814) (14.8438, -10.1879) (14.7885, -10.1947) (14.7332, -10.2019) (14.6782, -10.2094) (14.6233, -10.2173) (14.5686, -10.2256) (14.514, -10.2342) (14.4596, -10.2432) (14.4054, -10.2526) (14.3514, -10.2623) (14.2976, -10.2725) (14.2439, -10.283) (14.1905, -10.2938) (14.1372, -10.3051) (14.0841, -10.3167) (14.0313, -10.3288) (13.9786, -10.3412) (13.9262, -10.3541) (13.874, -10.3673) (13.822, -10.381) (13.7703, -10.3951) (13.7187, -10.4096) (13.6675, -10.4245) (13.6164, -10.4399) (13.5657, -10.4557) (13.5152, -10.472) (13.465, -10.4888) (13.4151, -10.506) (13.3655, -10.5237) (13.3161, -10.542) (13.2671, -10.5607) (13.2184, -10.5799) (13.17, -10.5996) (13.1221, -10.62) (13.0745, -10.641) (13.0274, -10.6627) (12.9808, -10.685) (12.9346, -10.7081) (12.889, -10.732) (12.8529, -10.7517) (12.8261, -10.7668) (12.8083, -10.777) (12.7994, -10.7821) knots -1 -1 -1 -1 -1 -1 -0.977778 -0.955556 -0.933333 -0.911111 -0.888889 -0.866667 -0.844444 -0.822222 -0.8 -0.777778 -0.755556 -0.733333 -0.711111 -0.688889 -0.666667 -0.644444 -0.622222 -0.6 -0.577778 -0.555556 -0.533333 -0.511111 -0.488889 -0.466667 -0.444444 -0.422222 -0.4 -0.377778 -0.355556 -0.333333 -0.311111 -0.288889 -0.266667 -0.244444 -0.222222 -0.2 -0.177778 -0.155556 -0.133333 -0.111111 -0.088889 -0.066667 -0.044444 -0.022222 0 0 0 0 0 0
  arc A29 (12.7994, -10.7821) -> (11.9393, -9.743) centre (0, -20.5) ccw
  spline S29 degree 5 poles (11.9393, -9.743) (11.9461, -9.7352) (11.9594, -9.7197) (11.9793, -9.6961) (12.0053, -9.6643) (12.0373, -9.624) (12.0686, -9.583) (12.0993, -9.5413) (12.1294, -9.4991) (12.1589, -9.4563) (12.1879, -9.413) (12.2164, -9.3692) (12.2444, -9.3249) (12.2719, -9.2803) (12.299, -9.2352) (12.3257, -9.1898) (12.352, -9.1439) (12.3778, -9.0978) (12.4033, -9.0512) (12.4283, -9.0043) (12.4529, -8.9571) (12.4772, -8.9095) (12.5011, -8.8616) (12.5246, -8.8134) (12.5477, -8.7649) (12.5705, -8.7161) (12.5929, -8.667) (12.615, -8.6176) (12.6367, -8.5679) (12.6581, -8.518) (12.6791, -8.4677) (12.6998, -8.4172) (12.7201, -8.3665) (12.7401, -8.3155) (12.7598, -8.2643) (12.7791, -8.2128) (12.7981, -8.161) (12.8168, -8.109) (12.8351, -8.0568) (12.8532, -8.0044) (12.8709, -7.9517) (12.8883, -7.8988) (12.9053, -7.8457) (12.9221, -7.7923) (12.9385, -7.7388) (12.9546, -7.685) (12.9673, -7.6419) (12.9766, -7.6094) (12.9828, -7.5877) (12.9859, -7.5768) knots 0 0 0 0 0 0 0.022222 0.044444 0.066667 0.088889 0.111111 0.133333 0.155556 0.177778 0.2 0.222222 0.244444 0.266667 0.288889 0.311111 0.333333 0.355556 0.377778 0.4 0.422222 0.444444 0.466667 0.488889 0.511111 0.533333 0.555556 0.577778 0.6 0.622222 0.644444 0.666667 0.688889 0.711111 0.733333 0.755556 0.777778 0.8 0.822222 0.844444 0.866667 0.888889 0.911111 0.933333 0.955556 0.977778 1 1 1 1 1 1
  arc A30 (12.9859, -7.5768) -> (12.6425, -7.2407) centre (0, -20.5) ccw
  spline S30 degree 5 poles (12.6425, -7.2407) (12.6317, -7.244) (12.6102, -7.2507) (12.5779, -7.2607) (12.535, -7.2743) (12.4816, -7.2915) (12.4284, -7.3091) (12.3754, -7.327) (12.3227, -7.3452) (12.2702, -7.3637) (12.2179, -7.3825) (12.1659, -7.4017) (12.114, -7.4212) (12.0625, -7.4409) (12.0112, -7.4611) (11.9601, -7.4815) (11.9093, -7.5022) (11.8587, -7.5233) (11.8084, -7.5447) (11.7584, -7.5665) (11.7086, -7.5886) (11.6591, -7.611) (11.6099, -7.6338) (11.561, -7.6569) (11.5124, -7.6804) (11.4641, -7.7042) (11.4161, -7.7284) (11.3684, -7.7529) (11.321, -7.7778) (11.274, -7.8031) (11.2273, -7.8287) (11.1809, -7.8547) (11.1349, -7.8812) (11.0893, -7.908) (11.0441, -7.9353) (10.9992, -7.9629) (10.9547, -7.991) (10.9107, -8.0195) (10.867, -8.0484) (10.8239, -8.0778) (10.7812, -8.1077) (10.739, -8.1381) (10.6974, -8.1691) (10.6565, -8.2007) (10.6161, -8.2329) (10.5765, -8.2657) (10.5452, -8.2924) (10.5221, -8.3128) (10.5068, -8.3265) (10.4992, -8.3333) knots -1 -1 -1 -1 -1 -1 -0.977778 -0.955556 -0.933333 -0.911111 -0.888889 -0.866667 -0.844444 -0.822222 -0.8 -0.777778 -0.755556 -0.733333 -0.711111 -0.688889 -0.666667 -0.644444 -0.622222 -0.6 -0.577778 -0.555556 -0.533333 -0.511111 -0.488889 -0.466667 -0.444444 -0.422222 -0.4 -0.377778 -0.355556 -0.333333 -0.311111 -0.288889 -0.266667 -0.244444 -0.222222 -0.2 -0.177778 -0.155556 -0.133333 -0.111111 -0.088889 -0.066667 -0.044444 -0.022222 0 0 0 0 0 0
  arc A31 (10.4992, -8.3333) -> (9.4419, -7.4957) centre (0, -20.5) ccw
  spline S31 degree 5 poles (9.4419, -7.4957) (9.4469, -7.4867) (9.4567, -7.4687) (9.4712, -7.4416) (9.4901, -7.4051) (9.513, -7.3589) (9.5351, -7.3123) (9.5565, -7.2652) (9.5772, -7.2176) (9.5971, -7.1696) (9.6165, -7.1212) (9.6352, -7.0725) (9.6534, -7.0234) (9.671, -6.974) (9.6882, -6.9243) (9.7048, -6.8743) (9.721, -6.824) (9.7367, -6.7734) (9.7519, -6.7226) (9.7666, -6.6715) (9.7809, -6.6202) (9.7947, -6.5686) (9.8081, -6.5168) (9.8211, -6.4648) (9.8337, -6.4125) (9.8458, -6.36) (9.8575, -6.3073) (9.8688, -6.2544) (9.8797, -6.2013) (9.8903, -6.148) (9.9004, -6.0945) (9.9101, -6.0409) (9.9194, -5.987) (9.9284, -5.9329) (9.937, -5.8787) (9.9452, -5.8243) (9.953, -5.7698) (9.9605, -5.715) (9.9676, -5.6602) (9.9743, -5.6051) (9.9807, -5.5499) (9.9867, -5.4945) (9.9923, -5.439) (9.9976, -5.3834) (10.0026, -5.3276) (10.0072, -5.2717) (10.0106, -5.2268) (10.0129, -5.1931) (10.0145, -5.1706) (10.0152, -5.1593) knots 0 0 0 0 0 0 0.022222 0.044444 0.066667 0.088889 0.111111 0.133333 0.155556 0.177778 0.2 0.222222 0.244444 0.266667 0.288889 0.311111 0.333333 0.355556 0.377778 0.4 0.422222 0.444444 0.466667 0.488889 0.511111 0.533333 0.555556 0.577778 0.6 0.622222 0.644444 0.666667 0.688889 0.711111 0.733333 0.755556 0.777778 0.8 0.822222 0.844444 0.866667 0.888889 0.911111 0.933333 0.955556 0.977778 1 1 1 1 1 1
  arc A32 (10.0152, -5.1593) -> (9.6095, -4.902) centre (0, -20.5) ccw